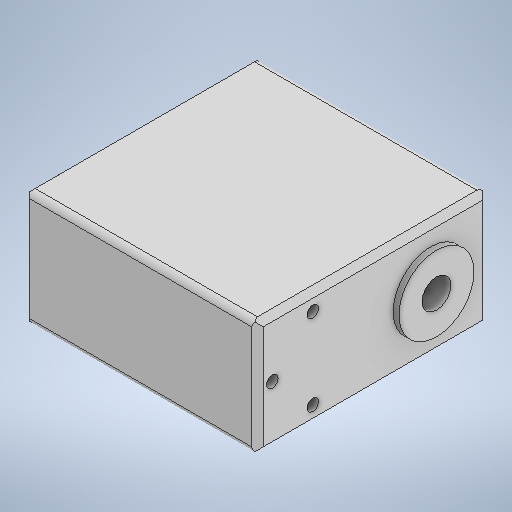
# Autodesk Inventor part: サーボパーツ1
Saved by Autodesk Inventor 2026.2 (Build 302298010, 298A)
## iProperties
Created: 2026-05-20
Part Number: サーボパーツ1
Material: 一般
Document SubType Name: Modeling
Designer: takan
Density: 1 g/cm^3
Appearance: 既定
Mass: 31.5001 g
Surface Area: 73.1435 cm^2
Volume: 31.5001 cm^3
Author: takan
Autodesk Inventor part; units mm, degrees
ref_plane "YZ Plane" through (0, 0, 0) normal (1, 0, 0) x (0, 1, 0)
ref_plane "XZ Plane" through (0, 0, 0) normal (0, 1, 0) x (-1, 0, 0)
ref_plane "XY Plane" through (0, 0, 0) normal (0, 0, 1) x (1, 0, 0)
sketch "スケッチ1" plane through (0, 0, 0) normal (0, 0, 1) x (1, 0, 0)
  line L0 (0, 0) -> (40.5, 0)
  line L1 (40.5, 0) -> (40.5, 20)
  line L2 (40.5, 20) -> (0, 20)
  line L3 (0, 20) -> (0, 0)
  dimension "d0" = 40.5
  dimension "d1" = 20
  constraints: 8 end point, 2 parallel, 1 horizontal, 1 perpendicular
  measures "d0" distance of L1.end L2.end
  measures "d1" distance of L0.end L1.end
extrude "押し出し1" add sketch "スケッチ1" along normal blind 40
sketch "スケッチ2" plane through (40.5, 0, 0) normal (1, 0, 0) x (0, 0, -1)
  circle A0 centre (-10, 10) radius 10
  line L0 (0, 0) -> (0, 20) projected
  line L1 (0, 10) -> (-40, 10)
  line L2 (-40, 0) -> (-40, 20) projected
  dimension "d4" = 20
  constraints: 3 midpoint, 2 end point, 1 horizontal alignment, 1 point on line, 2 other
hole "穴1" at (40.5, 10, 10) direction (-1, 0, 0) diameter 5 end through all
sketch "スケッチ3" plane through (40.5, 0, 0) normal (1, 0, 0) x (0, 0, -1)
  circle A0 centre (-10, 10) radius 6.5
  line L0 (0, 20) -> (0, 0) projected
  line L1 (0, 10) -> (-40, 10)
  line L2 (-40, 20) -> (-40, 0) projected
  circle A1 centre (-10, 10) radius 2.5 projected
  line L3 (-10, 12.5) -> (-10, 7.5)
  dimension "d12" = 13
  constraints: 4 end point, 3 midpoint, 2 point on circle, 1 centre point, 1 point on line, 1 vertical
  measures "d12" diameter of A0
extrude "押し出し2" add sketch "スケッチ3" along normal blind 1 contours L1 A1 A0 | A0 L1 A1
sketch "スケッチ4" plane through (0, 0, 0) normal (-1, 0, 0) x (0, 0, 1)
  circle A0 centre (10, 10) radius 2.5 projected
  line L0 (10, 12.5) -> (10, 7.5)
  line L1 (12.5, 10) -> (7.5, 10)
  circle A1 centre (10, 10) radius 6.5
  point P0 (0, 0)
  dimension "d15" = 13
  constraints: 4 end point, 4 point on circle, 1 centre point, 1 coincident, 1 perpendicular, 1 vertical
  measures "d15" diameter of A1
extrude "押し出し3" add sketch "スケッチ4" along normal blind 1
chamfer "面取り1" distance 1 angle 45 4 edges at (0, 20, 20) (40.5, 20, 20) (0, 0, 20) (40.5, 0, 20)
chamfer "面取り2" distance 1 angle 45 4 edges at (40.5, 10, 0) (0, 10, 0) (40.5, 10, 40) (0, 10, 40)
fillet "フィレット1" radius 1 4 edges at (20.25, 20, 40) (20.25, 0, 40) (20.25, 20, 0) (20.25, 0, 0)
sketch "スケッチ5" plane through (0, 1, 39) normal (-1, 0, 0) x (0, 0, 1)
  line L0 (-1.5, 16.5) -> (-16.5, 16.5)
  line L1 (-16.5, 16.5) -> (-16.5, 1.5)
  line L2 (-16.5, 1.5) -> (-1.5, 1.5)
  line L3 (-1.5, 1.5) -> (-1.5, 16.5)
  line L4 (0, 19) -> (-38, 19) projected
  line L5 (0, 18) -> (0, 0) projected
  point P0 (-39, -1)
  dimension "d25" = 15
  dimension "d26" = 2.5
  dimension "d27" = 15
  dimension "d45" = 1.5
  constraints: 8 end point, 2 parallel, 1 horizontal, 1 perpendicular
  measures "d25" distance of L2.end L0.start
  measures "d26" distance between parallel lines of L4 L0
  measures "d27" distance of L0.start L0.end
  measures "d45" distance between parallel lines of L3 L5
hole "穴2" at (0, 17.5, 22.5) at (0, 2.5, 22.5) at (0, 17.5, 37.5) at (0, 2.5, 37.5) direction (1, 0, 0) diameter 2 depth 8 tip angle 118
sketch "スケッチ6" plane through (40.5, 1, 39) normal (1, 0, 0) x (0, 0, -1)
  circle A0 centre (8.58, 9) radius 7
  line L0 (-1, 0) -> (-1, 18) projected
  line L1 (-1, 9) -> (38.1448, 9)
  line L2 (8.58, 16) -> (8.58, 2)
  line L3 (39, 0) -> (39, 18) projected
  point P0 (39, -1)
  point P1 (1.58, 9)
  dimension "d36" = 14
  dimension "d37" = 30.42
  constraints: 4 end point, 3 point on circle, 2 coincident, 2 midpoint, 2 point on line, 1 centre point, 1 horizontal
  measures "d36" diameter of A0
  measures "d37" distance between parallel lines of L3 L2
hole "穴3" at (40.5, 10, 37.42) at (40.5, 17, 30.42) at (40.5, 3, 30.42) direction (-1, 0, 0) diameter 2 depth 8 tip angle 118
